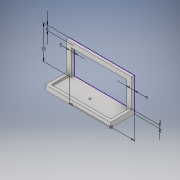
# Autodesk Inventor part: креплениедлякамерыниз
Saved by Autodesk Inventor 2019 (Build 230136000, 136)
## iProperties
Created: 2020-01-23
Part Number: креплениедлякамерыниз
Material: Типовые
Document SubType Name: Modeling
Designer: UlyaKZ
Density: 1 g/cm^3
Appearance: По умолчанию
Author: UlyaKZ
Autodesk Inventor part; units mm, degrees
ref_plane "YZ Plane" through (0, 0, 0) normal (1, 0, 0) x (0, 1, 0)
ref_plane "XZ Plane" through (0, 0, 0) normal (0, 1, 0) x (-1, 0, 0)
ref_plane "XY Plane" through (0, 0, 0) normal (0, 0, 1) x (1, 0, 0)
sketch "Эскиз1" plane through (0, 0, 0) normal (0, 0, 1) x (1, 0, 0)
  line L0 (0, 0) -> (68, 0)
  line L1 (68, 0) -> (68, 35)
  line L2 (68, 35) -> (0, 35)
  line L3 (0, 35) -> (0, 0)
  line L4 (5, 30) -> (63, 30)
  line L5 (63, 30) -> (63, 3)
  line L6 (63, 3) -> (5, 3)
  line L7 (5, 3) -> (5, 30)
  line L8 (5, 3) -> (0, 3)
  line L9 (63, 3) -> (68, 3)
  dimension "d0" = 5
  dimension "d1" = 5
  dimension "d2" = 5
  dimension "d3" = 3
  dimension "d4" = 68
  dimension "d5" = 35
  constraints: 20 end point, 7 perpendicular, 3 point on line, 2 horizontal
  measures "d0" distance between parallel lines of L4 L2
  measures "d1" distance between parallel lines of L3 L7
  measures "d2" distance between parallel lines of L1 L5
  measures "d3" distance between parallel lines of L0 L6
  measures "d4" distance between parallel lines of L1 L3
  measures "d5" distance between parallel lines of L0 L2
extrude "Выдавливание1" add sketch "Эскиз1" along normal blind 3 contours L3 L2 L1 L9 L5 L4 L7 L8
extrude "Выдавливание2" add sketch "Эскиз1" along normal blind 25 contours L3 L8 L6 L9 L1 L0
sketch "Эскиз2" plane through (0, 0, 0) normal (0, -1, 0) x (1, 0, 0)
  circle A0 centre (34, 12.5) radius 1
  line L0 (0, 0) -> (0, 25) projected
  line L1 (0, 25) -> (68, 25) projected
  point P0 (0, 12.5)
  point P1 (34, 25)
  dimension "d10" = 2
  constraints: 2 midpoint, 1 centre point, 1 horizontal alignment, 1 vertical alignment
  measures "d10" diameter of A0
extrude "Выдавливание3" cut sketch "Эскиз2" against normal up to next
sketch "Эскиз3" plane through (5, 3, 0) normal (0, 1, 0) x (1, 0, 0)
  line L0 (-5, -25) -> (63, -25) projected
  line L1 (-5, -3) -> (-5, -25)
  line L2 (-5, -25) -> (63, -25)
  line L3 (63, -25) -> (63, -3)
  line L4 (63, -3) -> (60, -3)
  line L5 (60, -3) -> (60, -22)
  line L6 (60, -22) -> (-2, -22)
  line L7 (-2, -22) -> (-2, -3)
  line L8 (-2, -3) -> (-5, -3)
  line L9 (58, -3) -> (63, -3) projected
  point P0 (-5, 0)
  point P1 (60.5, -3)
  dimension "d13" = 3
  dimension "d14" = 3
  dimension "d15" = 3
  constraints: 16 end point, 6 perpendicular, 2 vertical, 1 midpoint, 1 point on line
  measures "d13" distance between parallel lines of L1 L7
  measures "d14" distance between parallel lines of L5 L3
  measures "d15" distance between parallel lines of L0 L6
extrude "Выдавливание4" add sketch "Эскиз3" along normal blind 2
